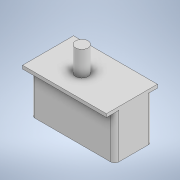
# Autodesk Inventor part: ESP8266 Feather
Saved by Autodesk Inventor 2021 (Build 250183000, 183)
## iProperties
Created: 2022-02-21
Part Number: ESP8266 Feather
Material: Generic
Document SubType Name: Modeling
Designer: maxsm
Density: 1 g/cm^3
Appearance: Default
Author: maxsm
Autodesk Inventor part; units mm, degrees
ref_plane "YZ Plane" through (0, 0, 0) normal (1, 0, 0) x (0, 1, 0)
ref_plane "XZ Plane" through (0, 0, 0) normal (0, 1, 0) x (-1, 0, 0)
ref_plane "XY Plane" through (0, 0, 0) normal (0, 0, 1) x (1, 0, 0)
sketch "Sketch1" plane through (0, 0, 0) normal (0, 1, 0) x (-1, 0, 0)
  line L0 (22.86, 11.43) -> (-22.86, 11.43)
  line L1 (-25.4, 8.89) -> (-25.4, -8.89)
  line L2 (-22.86, -11.43) -> (22.86, -11.43)
  line L3 (25.4, -8.89) -> (25.4, 8.89)
  line L4 (25.4, 11.43) -> (-25.4, -11.43) construction
  line L5 (-25.4, 11.43) -> (25.4, -11.43) construction
  circle A0 centre (22.86, 8.89) radius 1.27
  circle A1 centre (22.86, -8.89) radius 1.27
  circle A2 centre (-22.86, 9.525) radius 1.143
  circle A3 centre (-22.86, -9.525) radius 1.143
  arc A4 (25.4, 8.89) -> (22.86, 11.43) centre (22.86, 8.89) ccw
  arc A5 (22.86, -11.43) -> (25.4, -8.89) centre (22.86, -8.89) ccw
  arc A6 (-22.86, 11.43) -> (-25.4, 8.89) centre (-22.86, 8.89) ccw
  arc A7 (-25.4, -8.89) -> (-22.86, -11.43) centre (-22.86, -8.89) ccw
  point P0 (0, 0)
  dimension "d0" = 50.8
  dimension "d1" = 22.86
  dimension "d2" = 2.54
  dimension "d3" = 2.54
  dimension "d4" = 2.286
  dimension "d5" = 2.286
  dimension "d6" = 17.78
  dimension "d7" = 19.05
  dimension "d9" = 8.89
  dimension "d10" = 2.54
  dimension "d11" = 2.54
  dimension "d12" = 9.525
  dimension "d13" = 2.54
  dimension "d14" = 2.54
  dimension "d15" = 2.54
  constraints: 12 end point, 8 centre point, 8 point on circle, 8 point on line, 8 tangent, 3 equal radius, 2 midpoint, 2 parallel, 1 horizontal, 1 perpendicular
  measures "d0" distance of L5.end L4.end
  measures "d1" distance of L4.end L5.start
  measures "d2" diameter of A0
  measures "d3" diameter of A1
  measures "d4" diameter of A2
  measures "d5" diameter of A3
  measures "d6" distance of A1.centre A0.centre
  measures "d7" distance of A3.centre A2.centre
  measures "d9" vertical distance of A0.centre point (0, 0)
  measures "d10" distance from line of A0.centre L3
  measures "d11" distance from line of L3 A1.centre
  measures "d12" vertical distance of A2.centre point (0, 0)
  measures "d13" distance from line of L1 A3.centre
  measures "d14" distance from line of L1 A2.centre
  measures "d15" radius of A4
extrude "Extrusion1" add sketch "Sketch1" along normal blind 29
sketch "Sketch8" plane through (0, 29, 0) normal (0, 1, 0) x (1, 0, 0)
  circle A0 centre (-3.4, -2.54) radius 3.75
  line L0 (-25.4, 8.89) -> (-25.4, -8.89) projected
  point P0 (0, 0)
  dimension "d62" = 7.5
  dimension "d63" = 2.54
  dimension "d64" = 22
  constraints: 1 centre point
  measures "d62" diameter of A0
  measures "d63" vertical distance of point (0, 0) A0.centre
  measures "d64" distance from line of L0 A0.centre
extrude "Extrusion8" add sketch "Sketch8" along normal blind 15
sketch "Sketch9" plane through (0, 0, 0) normal (0, -1, 0) x (1, 0, 0)
  line L0 (-17.4, 8.93) -> (21.4, 8.93)
  line L1 (21.4, 8.93) -> (21.4, -8.93)
  line L2 (21.4, -8.93) -> (-17.4, -8.93)
  line L3 (-17.4, -8.93) -> (-17.4, 8.93)
  line L4 (-25.4, -8.89) -> (-25.4, 8.89) projected
  line L5 (25.4, 8.89) -> (25.4, -8.89) projected
  line L6 (-22.86, 11.43) -> (22.86, 11.43) projected
  line L7 (22.86, -11.43) -> (-22.86, -11.43) projected
  point P0 (0, 0)
  dimension "d67" = 8
  dimension "d68" = 4
  dimension "d69" = 2.5
  dimension "d70" = 2.5
  constraints: 8 end point, 2 parallel, 1 horizontal, 1 perpendicular
  measures "d67" distance between parallel lines of L4 L3
  measures "d68" distance between parallel lines of L5 L1
  measures "d69" distance between parallel lines of L0 L6
  measures "d70" distance between parallel lines of L7 L2
extrude "Extrusion9" add sketch "Sketch9" along normal blind 2
sketch "Sketch10" plane through (0, 29, 0) normal (0, 1, 0) x (1, 0, 0)
  line L0 (25.4, 14.43) -> (-25.4, 14.43)
  line L1 (-25.4, 14.43) -> (-25.4, -16.43)
  line L2 (-25.4, -16.43) -> (25.4, -16.43)
  line L3 (25.4, -16.43) -> (25.4, 14.43)
  line L4 (25.4, -8.89) -> (25.4, 8.89) projected
  line L5 (-25.4, 8.89) -> (-25.4, -8.89) projected
  line L6 (-22.86, -11.43) -> (22.86, -11.43) projected
  line L7 (22.86, 11.43) -> (-22.86, 11.43) projected
  point P0 (0, 0)
  point P1 (25.4, 0)
  point P2 (-25.4, -1)
  dimension "d73" = 5
  dimension "d74" = 3
  constraints: 8 end point, 2 midpoint, 2 parallel, 2 point on line, 1 horizontal, 1 perpendicular
  measures "d73" distance between parallel lines of L2 L6
  measures "d74" distance between parallel lines of L7 L0
extrude "Extrusion10" add sketch "Sketch10" against normal blind 2
body "Solid1"
